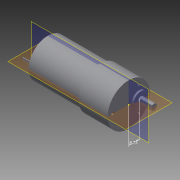
# Autodesk Inventor part: crouzet_motor
Saved by Autodesk Inventor 2015 (Build 190159000, 159)
## iProperties
Created: 2015-07-10
Part Number: crouzet_motor
Material: Generic
Description: insert part description/title
Document SubType Name: Modeling
Designer: francis
Mass: 160 g
Surface Area: 95.5468 cm^2
Volume: 59.9061 cm^3
Density: 2.67085 g/cm^3
Appearance: Default
Author: francis
Part Category: insert part category here and press enter to fill value
Autodesk Inventor part; units mm, degrees
ref_plane "YZ Plane" through (0, 0, 0) normal (1, 0, 0) x (0, 1, 0)
sketch "Sketch1" plane through (0, 0, 0) normal (0, 0, 1) x (1, 0, 0)
  line L0 (-37.0102, 0) -> (-37.0102, 16.1)
  line L1 (-37.0102, 16.1) -> (6.7898, 16.1)
  line L2 (6.7898, 16.1) -> (6.7898, 17.7)
  line L3 (6.7898, 17.7) -> (31.0898, 17.7)
  line L4 (31.0898, 17.7) -> (31.0898, 0)
  line L5 (31.0898, 0) -> (-37.0102, 0)
  line L6 (-42.8743, 0) -> (48.8507, 0) construction
  line L7 (0, 23.2775) -> (0, -29.7437) construction
  point P0 (0, 0)
  dimension "d0" = 16.1
  dimension "d1" = 68.1
  dimension "d2" = 24.3
  dimension "d3" = 17.7
  constraints: 16 end point, 5 perpendicular, 2 vertical, 1 horizontal
  measures "d0" distance of L0.start L0.end
  measures "d1" distance between parallel lines of L0 L4
  measures "d2" distance of L2.end L3.end
  measures "d3" distance between parallel lines of L5 L3
revolve "Revolution1" add sketch "Sketch1" angle 360 about axis through (-42.8743, 0, 0) along (1, 0, 0)
sketch "Sketch2" plane through (31.0898, 0, 0) normal (1, 0, 0) x (0, 0, -1)
  point P0 (0, 0)
  point P1 (0, 8.73)
  dimension "d5" = 8.73
  measures "d5" distance of point (0, 0) point (0, 8.73)
sketch "Sketch3" plane through (0, 0, 0) normal (0, 0, 1) x (1, 0, 0)
  line L0 (31.0898, 8.73) -> (43.5898, 8.73)
  line L1 (43.5898, 8.73) -> (43.5898, 11.23)
  line L2 (43.5898, 11.23) -> (32.5898, 11.23)
  line L3 (32.5898, 11.23) -> (32.5898, 14.73)
  line L4 (32.5898, 14.73) -> (31.0898, 14.73)
  line L5 (31.0898, 14.73) -> (31.0898, 8.73)
  line L6 (24.3312, 8.73) -> (72.9935, 8.73) construction
  line L7 (6.7898, -17.7) -> (6.7898, 17.7) construction
  point P0 (0, 0)
  dimension "d6" = 6
  dimension "d8" = 2.5
  dimension "d9" = 1.5
  dimension "d10" = 12.5
  constraints: 14 end point, 5 perpendicular, 2 point on line, 1 horizontal
  measures "d6" distance between parallel lines of L0 L4
  measures "d8" distance of L0.end L1.end
  measures "d9" distance of L3.end L4.end
  measures "d10" distance between parallel lines of L1 L5
revolve "Revolution2" add sketch "Sketch3" angle 360 about axis through (24.3312, 8.73, 0) along (1, 0, 0)
sketch "Sketch4" plane through (0, 0, 0) normal (0, 0, 1) x (1, 0, 0)
  line L0 (32.5898, 6.23) -> (43.5898, 6.23) projected
  line L1 (43.5898, 6.23) -> (34.0898, 6.23)
  line L2 (34.0898, 6.23) -> (34.0898, 7.23)
  line L3 (34.0898, 7.23) -> (43.5898, 7.23)
  line L4 (43.5898, 7.23) -> (43.5898, 6.23)
  point P0 (0, 0)
  dimension "d12" = 1
  dimension "d13" = 9.5
  constraints: 8 end point, 2 parallel, 1 horizontal, 1 perpendicular
  measures "d12" distance of L3.end L0.end
  measures "d13" distance of L2.end L3.end
extrude "Extrusion1" cut sketch "Sketch4" along normal mid plane 10
sketch "Sketch5" plane through (31.0898, 0, 0) normal (1, 0, 0) x (0, 0, -1)
  line L0 (0, -24.78) -> (0, 24.78) projected
  line L1 (-24.78, 0) -> (24.78, 0) projected
  point P0 (0, 0)
  point P1 (-10.25, 8.73)
  point P2 (10.25, 8.73)
  point P3 (0, -13.37)
  dimension "d16" = 20.5
  dimension "d17" = 8.73
  dimension "d18" = 22.1
  constraints: 1 point on line, 1 symmetric about line
  measures "d16" distance of point (-10.25, 8.73) point (10.25, 8.73)
  measures "d17" distance from line of L1 point (10.25, 8.73)
  measures "d18" vertical distance of point (0, -13.37) point (-10.25, 8.73)
hole "Hole1" at (31.0898, 8.73, 10.25) at (31.0898, 8.73, -10.25) at (31.0898, -13.37, 0) direction (-1, 0, 0) diameter 2.459 depth 4.5 thread size "M3x0.5" class "6H" standard "ISO Metric profile"
sketch "Sketch6" plane through (-37.0102, 0, 0) normal (-1, 0, 0) x (0, 0, 1)
  line L0 (0, 24.78) -> (0, -24.78) projected
  line L1 (-24.78, 0) -> (24.78, 0) projected
  line L2 (-1.4, 11.75) -> (1.4, 11.75)
  line L3 (1.4, 11.75) -> (1.4, 11.25)
  line L4 (1.4, 11.25) -> (-1.4, 11.25)
  line L5 (-1.4, 11.25) -> (-1.4, 11.75)
  line L6 (-1.4, -11.75) -> (1.4, -11.75)
  line L7 (1.4, -11.75) -> (1.4, -11.25)
  line L8 (1.4, -11.25) -> (-1.4, -11.25)
  line L9 (-1.4, -11.25) -> (-1.4, -11.75)
  point P0 (0, 0)
  point P1 (0, 11.25)
  point P2 (0, -11.25)
  dimension "d26" = 2.8
  dimension "d27" = 0.5
  dimension "d28" = 11.25
  constraints: 16 end point, 5 symmetric about line, 2 parallel, 1 horizontal, 1 midpoint, 1 perpendicular, 1 point on line
  measures "d26" distance of L3.end L4.end
  measures "d27" distance of L2.end L3.end
  measures "d28" distance between parallel lines of L1 L4
extrude "Extrusion2" add sketch "Sketch6" along normal blind 9.5
body "Solid1"
